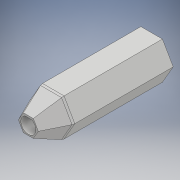
# Autodesk Inventor part: Bobinatge - acoplament eix
Saved by Autodesk Inventor 2019 (Build 230136000, 136)
## iProperties
Created: 2018-01-25
Part Number: Bobinatge - acoplament eix
Material: Genérico
Document SubType Name: Modeling
Designer: alber
Density: 1 g/cm^3
Appearance: Valor por defecto
Author: alber
Autodesk Inventor part; units mm, degrees
ref_plane "YZ Plane" through (0, 0, 0) normal (1, 0, 0) x (0, 1, 0)
ref_plane "XZ Plane" through (0, 0, 0) normal (0, 1, 0) x (-1, 0, 0)
ref_plane "XY Plane" through (0, 0, 0) normal (0, 0, 1) x (1, 0, 0)
sketch "Boceto11" plane through (0, 0, 0) normal (0, 1, 0) x (-1, 0, 0)
  line L0 (0, 0) -> (5.6, 0)
  line L1 (5.6, 0) -> (2.8, -4.8497)
  line L2 (2.8, -4.8497) -> (-2.8, -4.8497)
  line L3 (-2.8, -4.8497) -> (-5.6, 0)
  line L4 (-5.6, 0) -> (-2.8, 4.8497)
  line L5 (-2.8, 4.8497) -> (2.8, 4.8497)
  line L6 (2.8, 4.8497) -> (5.6, 0)
  line L7 (5.6, 0) -> (9.1, 0)
  line L8 (9.1, 0) -> (4.55, -7.8808)
  line L9 (4.55, -7.8808) -> (-4.55, -7.8808)
  line L10 (-4.55, -7.8808) -> (-9.1, 0)
  line L11 (-9.1, 0) -> (-4.55, 7.8808)
  line L12 (-4.55, 7.8808) -> (4.55, 7.8808)
  line L13 (4.55, 7.8808) -> (9.1, 0)
  dimension "d42" = 5.6
  dimension "d43" = 3.5
  constraints: 28 end point, 2 coincident, 1 horizontal, 1 point on line, 26 other
  measures "d42" distance of L0.start L0.end
  measures "d43" distance of L0.end L7.end
extrude "Extrusión10" add sketch "Boceto11" along normal blind 32
sketch "Boceto16" plane through (0, 0, 0) normal (0, -1, 0) x (1, 0, 0)
  line L0 (4.55, 7.8808) -> (9.1, 0) projected
  line L1 (9.1, 0) -> (4.55, -7.8808)
  line L2 (4.55, -7.8808) -> (-4.55, -7.8808)
  line L3 (-4.55, -7.8808) -> (-9.1, 0)
  line L4 (-9.1, 0) -> (-4.55, 7.8808)
  line L5 (-4.55, 7.8808) -> (4.55, 7.8808)
  line L6 (4.55, 7.8808) -> (9.1, 0)
  point P0 (0, 0)
  point P1 (0, 0)
  constraints: 12 end point, 1 coincident, 13 other
extrude "Extrusión14" add sketch "Boceto16" along normal blind 10 draft -23
sketch "Boceto19" plane through (0, -10, 0) normal (0, -1, 0) x (1, 0, 0)
  line L0 (-2.0993, 3.6361) -> (2.0993, 3.6361) projected
  line L1 (2.0993, -3.6361) -> (-2.0993, -3.6361) projected
  line L2 (2.0993, 3.6361) -> (4.1986, 0) projected
  line L3 (-4.55, -7.8808) -> (-2.0993, -3.6361) projected
  line L4 (-4.1986, 0) -> (-2.0993, 3.6361) projected
  arc A0 (-1.4491, 2.825) -> (1.4491, 2.825) centre (0, 0) ccw
  line L5 (0, 2.825) -> (-1.4491, 2.825)
  line L6 (0, 2.825) -> (1.4491, 2.825)
  constraints: 4 end point, 2 horizontal, 2 point on circle, 1 centre point
extrude "Extrusión16" cut sketch "Boceto19" against normal blind 15
sketch "Boceto20" plane through (0, 0, 0) normal (0, 1, 0) x (1, 0, 0)
  line L0 (-4.55, -7.8808) -> (-2.0993, -3.6361) projected
  line L1 (-2.7798, -4.8148) -> (-5.5597, 0)
  line L2 (-5.5597, 0) -> (-2.7798, 4.8148)
  line L3 (-2.7798, 4.8148) -> (2.7798, 4.8148)
  line L4 (2.7798, 4.8148) -> (5.5597, 0)
  line L5 (5.5597, 0) -> (2.7798, -4.8148)
  line L6 (2.7798, -4.8148) -> (-2.7798, -4.8148)
  point P0 (0, 0)
  point P1 (0, 0)
  constraints: 12 end point, 1 coincident, 1 point on line, 13 other
extrude "Extrusión17" add sketch "Boceto20" along normal blind 5
sketch "Boceto21" plane through (0, 32, 0) normal (0, 1, 0) x (1, 0, 0)
  line L0 (-5.6, 0) -> (-2.8, 4.8497)
  line L1 (-2.8, 4.8497) -> (2.8, 4.8497)
  line L2 (2.8, 4.8497) -> (5.6, 0)
  line L3 (5.6, 0) -> (2.8, -4.8497)
  line L4 (2.8, -4.8497) -> (-2.8, -4.8497)
  line L5 (-2.8, -4.8497) -> (-5.6, 0)
  line L6 (-2.8, -4.8497) -> (-5.6, 0) projected
  line L7 (-9.1, 0) -> (-4.55, -7.8808) projected
  line L8 (-4.55, -7.8808) -> (-9.1, 0)
  line L9 (-4.55, 7.8808) -> (-9.1, 0) projected
  line L10 (-9.1, 0) -> (-4.55, 7.8808)
  line L11 (4.55, 7.8808) -> (2.0993, 3.6361) projected
  line L12 (-4.55, 7.8808) -> (4.55, 7.8808)
  line L13 (4.55, -7.8808) -> (9.1, 0) projected
  line L14 (4.55, 7.8808) -> (9.1, 0)
  line L15 (9.1, 0) -> (4.55, -7.8808)
  line L16 (4.55, -7.8808) -> (-4.55, -7.8808)
  point P0 (0, 0)
  point P1 (0, 0)
  point P2 (0, 0)
  constraints: 24 end point, 6 equal length, 2 coincident, 1 horizontal, 1 point on line, 11 other
chamfer "Chaflán1" distance 0.5 angle 45 6 edges at (0, 0, -7.8808) (-6.825, 0, -3.9404) (6.825, 0, -3.9404) (-6.825, 0, 3.9404) (0, 0, 7.8808) (6.825, 0, 3.9404)
extrude "Extrusión19" add sketch "Boceto21" along normal blind 10
